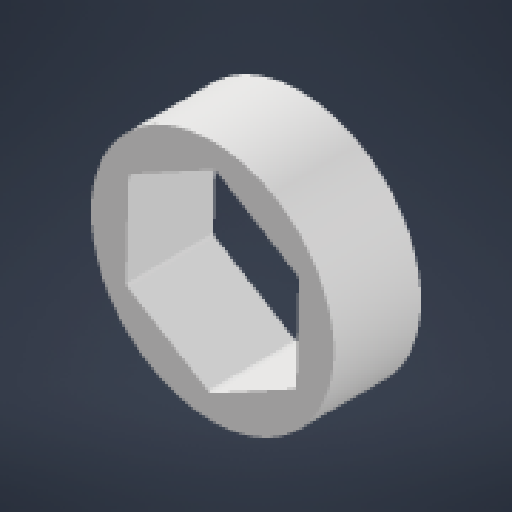
# Autodesk Inventor part: Servo_Spacer
Saved by Autodesk Inventor 2024.2 (Build 282272000, 272)
## iProperties
Created: 2024-03-30
Part Number: Servo_Spacer
Material: Generic
Document SubType Name: Modeling
Designer: warm
Density: 1 g/cm^3
Appearance: Default
Author: warm
Autodesk Inventor part; units mm, degrees
ref_plane "YZ Plane" through (0, 0, 0) normal (1, 0, 0) x (0, 1, 0)
ref_plane "XZ Plane" through (0, 0, 0) normal (0, 1, 0) x (-1, 0, 0)
sketch "Sketch1" plane through (0, 0, 0) normal (0, 0, 1) x (1, 0, 0)
  circle A0 centre (0, 0) radius 1.525
  line L0 (3.3712, -2.153) -> (-0.0331, -3.9999)
  arc A1 (-0.1789, -3.996) -> (-0.0331, -3.9999) centre (0, 0) ccw
  line L1 (-0.1789, -3.996) -> (-3.4805, -1.9713)
  arc A2 (-3.5501, -1.843) -> (-3.4805, -1.9713) centre (0, 0) ccw
  line L2 (-3.5501, -1.843) -> (-3.4474, 2.0286)
  arc A3 (-3.3712, 2.153) -> (-3.4474, 2.0286) centre (0, 0) ccw
  line L3 (-3.3712, 2.153) -> (0.0331, 3.9999)
  arc A4 (0.1789, 3.996) -> (0.0331, 3.9999) centre (0, 0) ccw
  line L4 (0.1789, 3.996) -> (3.4805, 1.9713)
  arc A5 (3.5501, 1.843) -> (3.4805, 1.9713) centre (0, 0) ccw
  line L5 (3.5501, 1.843) -> (3.4474, -2.0286)
  arc A6 (3.3712, -2.153) -> (3.4474, -2.0286) centre (0, 0) ccw
  circle A7 centre (0, 0) radius 5
  point P0 (0, 0)
  dimension "d0" = 10
  constraints: 12 end point, 12 point on circle, 8 centre point, 1 coincident, 32 other
  measures "d0" diameter of A7
ref_plane "Work Plane1" through (-10.187, -10.187, 3.6) normal (0, 0, -1) x (0.5228, 0.8525, 0)
extrude "Extrusion1" add sketch "Sketch1" along normal up to surface (3.6 mm away) contours A7
body "Solid1"
